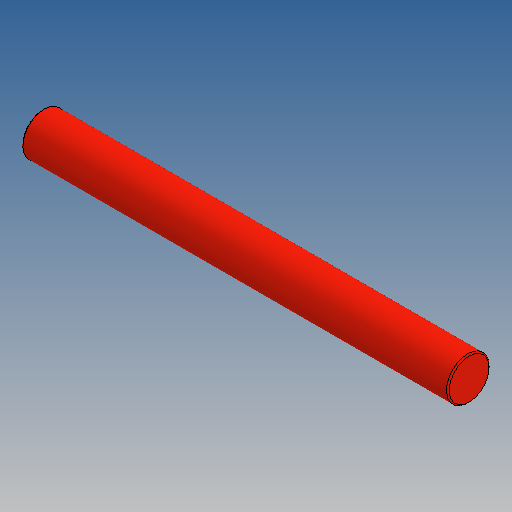
# Autodesk Inventor part: 21462-Red
Saved by Autodesk Inventor 2025.1 (Build 291241000, 241)
## iProperties
Created: 2014-06-03
Part Number: 21462-Red
Material: ABS Plastic
Document SubType Name: Modeling
Designer: D. Kohfeld
Appearance: Red
Mass: 0.272756 g
Surface Area: 3.36912 cm^2
Volume: 0.257317 cm^3
Density: 1.06 g/cm^3
Author: D. Kohfeld
Autodesk Inventor part; units mm, degrees
ref_plane "YZ Plane" through (0, 0, 0) normal (1, 0, 0) x (0, 1, 0)
ref_plane "XZ Plane" through (0, 0, 0) normal (0, 1, 0) x (-1, 0, 0)
ref_plane "XY Plane" through (0, 0, 0) normal (0, 0, 1) x (1, 0, 0)
sketch "Sketch1" plane through (0, 0, 0) normal (1, 0, 0) x (0, 1, 0)
  circle A0 centre (0, 0) radius 1.6
  dimension "d26" = 3.2
  constraints: 1 centre point, 1 coincident
  measures "d26" diameter of A0
extrude "Extrusion7" add sketch "Sketch1" along normal mid plane 32
fillet "Fillet2" radius 0.1 2 edges at (16, -1.6, 0) (-16, -1.6, 0)
equation "\"d26\" = rd"
equation "\"d27\" = 4 * lu"
equation "\"rd\" = 3.2"
equation "\"lu\" = 8"
body "Solid2"
